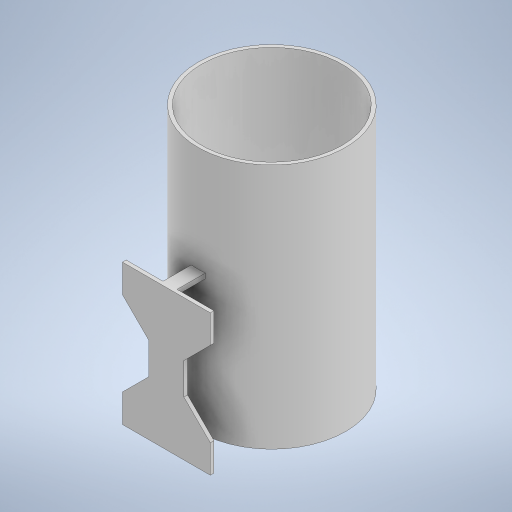
# Autodesk Inventor part: solo_rurka
Saved by Autodesk Inventor 2023 (Build 270158000, 158)
## iProperties
Created: 2023-03-15
Part Number: solo_rurka
Material: Ogólny
Document SubType Name: Modeling
Designer: kamil
Density: 1 g/cm^3
Appearance: Domyślna
Author: kamil
Autodesk Inventor part; units mm, degrees
ref_plane "YZ Plane" through (0, 0, 0) normal (1, 0, 0) x (0, 1, 0)
ref_plane "XZ Plane" through (0, 0, 0) normal (0, 1, 0) x (-1, 0, 0)
ref_plane "XY Plane" through (0, 0, 0) normal (0, 0, 1) x (1, 0, 0)
sketch "Szkic1" plane through (0, 0, 0) normal (0, 1, 0) x (-1, 0, 0)
  circle A0 centre (0, -30) radius 20
  line L0 (12.5, 0) -> (-12.5, 0)
  line L1 (-12.5, 0) -> (-12.5, -1.05)
  line L2 (-12.5, -1.05) -> (12.5, -1.05)
  line L3 (12.5, -1.05) -> (12.5, 0)
  circle A1 centre (0, -30) radius 21
  line L4 (-2, -9.0955) -> (2, -9.0955)
  line L5 (2, -9.0955) -> (2, -1.05)
  line L6 (2, -1.05) -> (-2, -1.05)
  line L7 (-2, -1.05) -> (-2, -9.0955)
  point P0 (0, 0)
  point P1 (0, -1.05)
  point P2 (0, 0)
  point P3 (0, -9.0955)
  dimension "d15" = 40
  dimension "d16" = 25
  dimension "d17" = 1.05
  dimension "d18" = 30
  dimension "d19" = 1
  dimension "d20" = 4
  constraints: 16 end point, 4 parallel, 3 midpoint, 3 vertical alignment, 2 horizontal, 2 perpendicular, 1 centre point, 1 coincident, 1 horizontal alignment, 1 point on line, 3 other
  measures "d15" diameter of A0
  measures "d16" distance of L0.start L0.end
  measures "d17" distance of L2.end L0.start
  measures "d18" distance of point (0, 0) A0.centre
  measures "d20" distance of L4.start L4.end
extrude "Wyciągnięcie proste1" add sketch "Szkic1" along normal blind 40 contours L3 L2 L1 L0
extrude "Extrusion2" add sketch "Szkic1" along normal blind 1.2 contours L5 A1 L7 L2 | L4 A1 picked at (0.2225, -9.0672)
sketch "Sketch2" plane through (-12.5, 0, 0) normal (0, 0, 1) x (1, 0, 0)
  line L0 (25, 40) -> (0, 40) projected
  line L1 (25, 0) -> (25, 40) projected
  line L2 (0, 40) -> (25, 40)
  line L3 (25, 40) -> (25, 32)
  line L4 (25, 32) -> (13, 20)
  line L5 (25, 8) -> (25, 0)
  line L6 (0, 0) -> (0, 40) projected
  line L7 (25, 0) -> (0, 0)
  line L8 (0, 0) -> (0, 8)
  line L9 (12, 20) -> (0, 32)
  line L10 (0, 32) -> (0, 40)
  line L11 (17.5, 60) -> (27.5, 60) construction
  line L12 (0, 20) -> (25, 20) construction
  line L13 (0, 8) -> (12, 20)
  line L14 (25, 8) -> (13, 20)
  line L15 (12.5, 40) -> (12.5, 0) construction
  line L16 (0, 40) -> (25, 40) construction
  line L17 (0, 0) -> (25, 0) construction
  line L18 (7.5, 15.5) -> (7.5, 24.5)
  line L19 (17.5, 15.5) -> (17.5, 24.5)
  point P0 (0, 32)
  dimension "d24" = 45
  dimension "d26" = 8
  dimension "d48" = 8
  dimension "d49" = 10
  constraints: 29 end point, 9 point on line, 4 perpendicular, 3 midpoint, 2 vertical, 1 horizontal alignment, 1 parallel, 3 other
  measures "d24" angle to the sketch x axis of L4
  measures "d26" distance of L1.end L3.end
  measures "d48" distance of L5.start L1.start
  measures "d49" distance between parallel lines of L19 L18
extrude "Extrusion3" cut sketch "Sketch2" against normal blind 1.2 contours L1 L14 L19 L4 | L9 L18 L13 L6
sketch "Sketch4" plane through (0, 0, 0) normal (1, 0, 0) x (0, 1, 0)
  line L0 (1.2, -9.0955) -> (1.2, -1.05) projected
  line L1 (38.6, -9.0955) -> (38.6, -1.05)
  line L2 (32, -1.05) -> (40, -1.05) projected
  line L3 (40, -1.05) -> (40, -9.0955)
  line L4 (1.2, -2.7471) -> (1.2, -1.05)
  line L5 (1.2, -1.05) -> (1.2, -9.0955) projected
  line L6 (32, -1.05) -> (24.5, -1.05) projected
  line L7 (40, -9.0955) -> (38.6, -9.0955)
  line L8 (32, -1.05) -> (40, -1.05) projected
  point P0 (0, 0)
  point P1 (1.2, -14.3431)
  point P2 (20, -1.05)
  point P3 (25, -1.05)
  dimension "d32" = 1.4
  constraints: 8 end point, 2 parallel, 1 collinear, 1 horizontal alignment, 1 perpendicular, 1 point on line
  measures "d32" distance between parallel lines of L3 L1
extrude "Extrusion4" add sketch "Sketch4" along normal mid plane 4
extrude "Extrusion5" add sketch "Szkic1" along normal blind 70 contours L4 A1 | A1 L4
extrude "Wyciągnięcie proste6" cut sketch "Szkic1" along normal blind 70 contours A0
equation "\"d26\" = d48"
equation "\"d35\" = d20"
